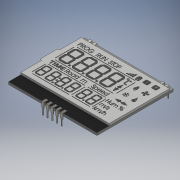
# Autodesk Inventor part: DF700543-05
Saved by Autodesk Inventor 2018 (Build 220112000, 112)
## iProperties
Created: 2018-02-18
Part Number: DF700543-05
Material: Generic
Document SubType Name: Modeling
Designer: danil
Density: 1 g/cm^3
Appearance: Default
Mass: 10.2861 g
Surface Area: 134.254 cm^2
Volume: 10.2861 cm^3
Author: danil
Autodesk Inventor part; units mm, degrees
(part 1 of 3)
ref_plane "YZ Plane" through (0, 0, 0) normal (1, 0, 0) x (0, 1, 0)
ref_plane "XZ Plane" through (0, 0, 0) normal (0, 1, 0) x (-1, 0, 0)
ref_plane "XY Plane" through (0, 0, 0) normal (0, 0, 1) x (1, 0, 0)
sketch "Sketch1" plane through (0, 0, 0) normal (0, 0, 1) x (1, 0, 0)
  line L0 (-23.765, -20.5) -> (23.765, -20.5)
  line L1 (23.765, -20.5) -> (23.765, 20.5)
  line L2 (23.765, 20.5) -> (-23.765, 20.5)
  line L3 (-23.765, 20.5) -> (-23.765, -20.5)
  line L4 (-23.765, -20.5) -> (23.765, 20.5) construction
  line L5 (23.765, -20.5) -> (-23.765, 20.5) construction
  arc A0 (-24.7705, -1.85) -> (-23.765, -2.75) centre (-23.865, -1.85) ccw
  arc A1 (-23.765, 7.25) -> (-24.7705, 6.35) centre (-23.865, 6.35) ccw
  line L6 (-24.7705, 6.35) -> (-24.7705, -1.85)
  point P0 (0, 0)
  point P1 (-24.765, -1.85)
  point P2 (-24.765, 6.35)
  dimension "d0" = 47.53
  dimension "d1" = 41
  constraints: 14 end point, 4 point on circle, 2 centre point, 2 coincident, 2 midpoint, 2 parallel, 2 point on line, 1 horizontal, 1 perpendicular
  measures "d0" distance of L2.end L1.end
  measures "d1" distance of L1.end L0.end
extrude "Extrusion1" add sketch "Sketch1" along normal blind 1.2
sketch "Sketch2" plane through (0, 0, 1.2) normal (0, 0, 1) x (1, 0, 0)
  line L0 (-23.765, 20.5) -> (-23.765, -20.5) projected
  line L1 (23.765, -20.5) -> (23.765, 20.5) projected
  line L2 (-23.765, 18.5) -> (23.765, 18.5)
  line L3 (23.765, 18.5) -> (23.765, -14)
  line L4 (23.765, -14) -> (-23.765, -14)
  line L5 (-23.765, -14) -> (-23.765, 18.5)
  arc A0 (-23.765, 7.25) -> (-24.7705, 6.35) centre (-23.865, 6.35) ccw projected
  line L6 (-24.7705, 6.35) -> (-24.7705, -1.85) projected
  arc A1 (-24.7705, -1.85) -> (-23.765, -2.75) centre (-23.865, -1.85) ccw projected
  line L7 (-23.765, -20.5) -> (23.765, -20.5) projected
  line L8 (23.765, 20.5) -> (-23.765, 20.5) projected
  dimension "d13" = 6.5
  dimension "d14" = 2
  constraints: 8 end point, 2 parallel, 2 point on line, 1 horizontal, 1 perpendicular
  measures "d13" distance between parallel lines of L4 L7
  measures "d14" distance between parallel lines of L8 L2
extrude "Extrusion2" add sketch "Sketch2" along normal blind 1.2 separate body contours L2 L1 L4 L0 | L0 A1 L6 A0
sketch "Sketch3" plane through (0, 0, 2.4) normal (0, 0, 1) x (1, 0, 0)
  line L0 (-19.2352, 12.1702) -> (-15.8959, 12.1702)
  line L1 (-15.8959, 12.1702) -> (-15.3617, 11.6361)
  line L2 (-15.3617, 11.6361) -> (-15.8375, 11.1603)
  line L3 (-15.8375, 11.1603) -> (-19.2759, 11.1603)
  line L4 (-19.2759, 11.1603) -> (-19.7605, 11.6449)
  line L5 (-19.7605, 11.6449) -> (-19.2352, 12.1702)
  line L6 (-19.8454, 11.56) -> (-19.3492, 11.0639)
  line L7 (-19.3492, 11.0639) -> (-19.3492, 7.616)
  line L8 (-19.3492, 7.616) -> (-19.8657, 7.0995)
  line L9 (-19.8657, 7.0995) -> (-20.3591, 7.5929)
  line L10 (-20.3591, 7.5929) -> (-20.3591, 11.0462)
  line L11 (-20.3591, 11.0462) -> (-19.8454, 11.56)
  line L12 (-15.2769, 11.5512) -> (-15.7818, 11.0462)
  line L13 (-15.7818, 11.0462) -> (-15.7818, 7.6242)
  line L14 (-15.7818, 7.6242) -> (-15.2572, 7.0995)
  line L15 (-15.2572, 7.0995) -> (-14.7719, 7.5848)
  line L16 (-14.7719, 7.5848) -> (-14.7719, 11.0462)
  line L17 (-14.7719, 11.0462) -> (-15.2769, 11.5512)
  line L18 (-19.7809, 7.0146) -> (-19.2759, 7.5196)
  line L19 (-19.2759, 7.5196) -> (-15.847, 7.5196)
  line L20 (-15.847, 7.5196) -> (-15.342, 7.0146)
  line L21 (-15.342, 7.0146) -> (-15.847, 6.5097)
  line L22 (-15.847, 6.5097) -> (-19.2759, 6.5097)
  line L23 (-19.2759, 6.5097) -> (-19.7809, 7.0146)
  line L24 (-19.8657, 6.9298) -> (-20.3591, 6.4364)
  line L25 (-20.3591, 6.4364) -> (-20.3591, 3.0156)
  line L26 (-20.3591, 3.0156) -> (-19.8379, 2.4943)
  line L27 (-19.8379, 2.4943) -> (-19.3492, 2.983)
  line L28 (-19.3492, 2.983) -> (-19.3492, 6.4133)
  line L29 (-19.3492, 6.4133) -> (-19.8657, 6.9298)
  line L30 (-19.753, 2.4095) -> (-19.2759, 1.9324)
  line L31 (-19.2759, 1.9324) -> (-15.847, 1.9324)
  line L32 (-15.847, 1.9324) -> (-15.3739, 2.4054)
  line L33 (-15.3739, 2.4054) -> (-15.9108, 2.9423)
  line L34 (-15.9108, 2.9423) -> (-19.2202, 2.9423)
  line L35 (-19.2202, 2.9423) -> (-19.753, 2.4095)
  line L36 (-15.2891, 2.4903) -> (-15.7818, 2.983)
  line L37 (-15.7818, 2.983) -> (-15.7818, 6.4051)
  line L38 (-15.7818, 6.4051) -> (-15.2572, 6.9298)
  line L39 (-15.2572, 6.9298) -> (-14.7719, 6.4445)
  line L40 (-14.7719, 6.4445) -> (-14.7719, 3.0075)
  line L41 (-14.7719, 3.0075) -> (-15.2891, 2.4903)
  line L42 (-14.3647, 2.8446) -> (-13.4606, 2.8446)
  line L43 (-13.4606, 2.8446) -> (-13.4606, 1.9405)
  line L44 (-13.4606, 1.9405) -> (-14.3647, 1.9405)
  line L45 (-14.3647, 1.9405) -> (-14.3647, 2.8446)
  line L46 (-7.9514, 7.0995) -> (-7.4661, 7.5848)
  line L47 (-8.0363, 7.0146) -> (-8.5412, 6.5097)
  line L48 (-7.4661, 7.5848) -> (-7.4661, 11.0462)
  line L49 (-8.4761, 11.0462) -> (-8.4761, 7.6242)
  line L50 (-7.4661, 11.0462) -> (-7.9711, 11.5512)
  line L51 (-8.056, 11.6361) -> (-8.5318, 11.1603)
  line L52 (-8.4761, 7.6242) -> (-7.9514, 7.0995)
  line L53 (-7.4661, 6.4445) -> (-7.4661, 3.0075)
  line L54 (-8.4761, 2.983) -> (-8.4761, 6.4051)
  line L55 (-8.6051, 2.9423) -> (-11.9145, 2.9423)
  line L56 (-11.9701, 1.9324) -> (-8.5412, 1.9324)
  line L57 (-12.4473, 2.4095) -> (-11.9701, 1.9324)
  line L58 (-11.9145, 2.9423) -> (-12.4473, 2.4095)
  line L59 (-12.5321, 2.4943) -> (-12.0434, 2.983)
  line L60 (-8.5412, 6.5097) -> (-11.9701, 6.5097)
  line L61 (-11.9701, 7.5196) -> (-8.5412, 7.5196)
  line L62 (-12.0434, 2.983) -> (-12.0434, 6.4133)
  line L63 (-11.9701, 6.5097) -> (-12.4751, 7.0146)
  line L64 (-12.4751, 7.0146) -> (-11.9701, 7.5196)
  line L65 (-13.0534, 6.4364) -> (-13.0534, 3.0156)
  line L66 (-13.0534, 3.0156) -> (-12.5321, 2.4943)
  line L67 (-8.4761, 6.4051) -> (-7.9514, 6.9298)
  line L68 (-8.5412, 7.5196) -> (-8.0363, 7.0146)
  line L69 (-7.9514, 6.9298) -> (-7.4661, 6.4445)
  line L70 (-8.0682, 2.4054) -> (-8.6051, 2.9423)
  line L71 (-8.5412, 1.9324) -> (-8.0682, 2.4054)
  line L72 (-7.4661, 3.0075) -> (-7.9833, 2.4903)
  line L73 (-7.9833, 2.4903) -> (-8.4761, 2.983)
  line L74 (-7.9711, 11.5512) -> (-8.4761, 11.0462)
  line L75 (-11.9294, 12.1702) -> (-8.5901, 12.1702)
  line L76 (-8.5901, 12.1702) -> (-8.056, 11.6361)
  line L77 (-8.5318, 11.1603) -> (-11.9701, 11.1603)
  line L78 (-11.9701, 11.1603) -> (-12.4547, 11.6449)
  line L79 (-12.4547, 11.6449) -> (-11.9294, 12.1702)
  line L80 (-12.5396, 11.56) -> (-12.0434, 11.0639)
  line L81 (-12.0434, 11.0639) -> (-12.0434, 7.616)
  line L82 (-12.0434, 7.616) -> (-12.56, 7.0995)
  line L83 (-12.56, 6.9298) -> (-13.0534, 6.4364)
  line L84 (-12.56, 7.0995) -> (-13.0534, 7.5929)
  line L85 (-13.0534, 7.5929) -> (-13.0534, 11.0462)
  line L86 (-13.0534, 11.0462) -> (-12.5396, 11.56)
  line L87 (-12.0434, 6.4133) -> (-12.56, 6.9298)
  line L88 (-0.6375, 7.0995) -> (-0.1522, 7.5848)
  line L89 (-0.7223, 7.0146) -> (-1.2273, 6.5097)
  line L90 (-0.1522, 7.5848) -> (-0.1522, 11.0462)
  line L91 (-1.1622, 11.0462) -> (-1.1622, 7.6242)
  line L92 (-0.1522, 11.0462) -> (-0.6572, 11.5512)
  line L93 (-0.742, 11.6361) -> (-1.2178, 11.1603)
  line L94 (-1.1622, 7.6242) -> (-0.6375, 7.0995)
  line L95 (-0.1522, 6.4445) -> (-0.1522, 3.0075)
  line L96 (-1.1622, 2.983) -> (-1.1622, 6.4051)
  line L97 (-1.2911, 2.9423) -> (-4.6005, 2.9423)
  line L98 (-4.6562, 1.9324) -> (-1.2273, 1.9324)
  line L99 (-5.1333, 2.4095) -> (-4.6562, 1.9324)
  line L100 (-4.6005, 2.9423) -> (-5.1333, 2.4095)
  line L101 (-5.2182, 2.4943) -> (-4.7295, 2.983)
  line L102 (-1.2273, 6.5097) -> (-4.6562, 6.5097)
  line L103 (-4.6562, 7.5196) -> (-1.2273, 7.5196)
  line L104 (-4.7295, 2.983) -> (-4.7295, 6.4133)
  line L105 (-4.6562, 6.5097) -> (-5.1612, 7.0146)
  line L106 (-5.1612, 7.0146) -> (-4.6562, 7.5196)
  line L107 (-5.7395, 6.4364) -> (-5.7395, 3.0156)
  line L108 (-5.7395, 3.0156) -> (-5.2182, 2.4943)
  line L109 (-1.1622, 6.4051) -> (-0.6375, 6.9298)
  line L110 (-1.2273, 7.5196) -> (-0.7223, 7.0146)
  line L111 (-0.6375, 6.9298) -> (-0.1522, 6.4445)
  line L112 (-0.7543, 2.4054) -> (-1.2911, 2.9423)
  line L113 (-1.2273, 1.9324) -> (-0.7543, 2.4054)
  line L114 (-0.1522, 3.0075) -> (-0.6694, 2.4903)
  line L115 (-0.6694, 2.4903) -> (-1.1622, 2.983)
  line L116 (-0.6572, 11.5512) -> (-1.1622, 11.0462)
  line L117 (-4.6155, 12.1702) -> (-1.2762, 12.1702)
  line L118 (-1.2762, 12.1702) -> (-0.742, 11.6361)
  line L119 (-1.2178, 11.1603) -> (-4.6562, 11.1603)
  line L120 (-4.6562, 11.1603) -> (-5.1408, 11.6449)
  line L121 (-5.1408, 11.6449) -> (-4.6155, 12.1702)
  line L122 (-5.2257, 11.56) -> (-4.7295, 11.0639)
  line L123 (-4.7295, 11.0639) -> (-4.7295, 7.616)
  line L124 (-4.7295, 7.616) -> (-5.246, 7.0995)
  line L125 (-5.246, 6.9298) -> (-5.7395, 6.4364)
  line L126 (-5.246, 7.0995) -> (-5.7395, 7.5929)
  line L127 (-5.7395, 7.5929) -> (-5.7395, 11.0462)
  line L128 (-5.7395, 11.0462) -> (-5.2257, 11.56)
  line L129 (-4.7295, 6.4133) -> (-5.246, 6.9298)
  line L130 (-7.0426, 2.8446) -> (-6.1386, 2.8446)
  line L131 (-6.1386, 2.8446) -> (-6.1386, 1.9405)
  line L132 (-6.1386, 1.9405) -> (-7.0426, 1.9405)
  line L133 (-7.0426, 1.9405) -> (-7.0426, 2.8446)
  line L134 (6.6113, 7.0995) -> (7.0965, 7.5848)
  line L135 (7.0965, 7.5848) -> (7.0965, 11.0462)
  line L136 (6.0866, 11.0462) -> (6.0866, 7.6242)
  line L137 (2.5925, 7.5196) -> (6.0214, 7.5196)
  line L138 (6.0866, 7.6242) -> (6.6113, 7.0995)
  line L139 (6.0214, 7.5196) -> (6.5264, 7.0146)
  line L140 (2.5192, 11.0639) -> (2.5192, 7.616)
  line L141 (1.5093, 7.5929) -> (1.5093, 11.0462)
  line L142 (2.5192, 7.616) -> (2.0027, 7.0995)
  line L143 (2.0876, 7.0146) -> (2.5925, 7.5196)
  line L144 (2.0027, 7.0995) -> (1.5093, 7.5929)
  line L145 (6.5264, 7.0146) -> (6.0214, 6.5097)
  line L146 (1.5093, 6.4364) -> (1.5093, 3.0156)
  line L147 (1.5093, 3.0156) -> (2.0306, 2.4943)
  line L148 (2.5192, 2.983) -> (2.5192, 6.4133)
  line L149 (6.0214, 6.5097) -> (2.5925, 6.5097)
  line L150 (2.0306, 2.4943) -> (2.5192, 2.983)
  line L151 (2.6482, 2.9423) -> (2.1154, 2.4095)
  line L152 (2.1154, 2.4095) -> (2.5925, 1.9324)
  line L153 (6.0866, 6.4051) -> (6.6113, 6.9298)
  line L154 (6.6113, 6.9298) -> (7.0965, 6.4445)
  line L155 (6.0866, 2.983) -> (6.0866, 6.4051)
  line L156 (7.0965, 6.4445) -> (7.0965, 3.0075)
  line L157 (2.5925, 1.9324) -> (6.0214, 1.9324)
  line L158 (5.9576, 2.9423) -> (2.6482, 2.9423)
  line L159 (2.0027, 6.9298) -> (1.5093, 6.4364)
  line L160 (2.5192, 6.4133) -> (2.0027, 6.9298)
  line L161 (2.5925, 6.5097) -> (2.0876, 7.0146)
  line L162 (1.5093, 11.0462) -> (2.0231, 11.56)
  line L163 (2.0231, 11.56) -> (2.5192, 11.0639)
  line L164 (2.5925, 11.1603) -> (2.1079, 11.6449)
  line L165 (6.0309, 11.1603) -> (2.5925, 11.1603)
  line L166 (7.0965, 11.0462) -> (6.5916, 11.5512)
  line L167 (6.5916, 11.5512) -> (6.0866, 11.0462)
  line L168 (6.5067, 11.6361) -> (6.0309, 11.1603)
  line L169 (5.9726, 12.1702) -> (6.5067, 11.6361)
  line L170 (2.6333, 12.1702) -> (5.9726, 12.1702)
  line L171 (2.1079, 11.6449) -> (2.6333, 12.1702)
  line L172 (6.4945, 2.4054) -> (5.9576, 2.9423)
  line L173 (6.0214, 1.9324) -> (6.4945, 2.4054)
  line L174 (6.5794, 2.4903) -> (6.0866, 2.983)
  line L175 (7.0965, 3.0075) -> (6.5794, 2.4903)
  line L176 (14.4675, 11.3639) -> (16.3084, 9.9795) construction
  line L177 (16.3084, 9.9795) -> (14.9887, 8.0409) construction
  spline S0 degree 2 poles (14.4675, 11.3639) (16.3084, 9.9795) (14.9887, 8.0409) knots 1 1 1 2 2 2
  line L178 (14.9887, 8.0409) -> (12.6861, 9.6083) construction
  line L179 (12.6861, 9.6083) -> (14.605, 9.7205) construction
  line L180 (14.605, 9.7205) -> (14.1661, 10.7205) construction
  spline S1 degree 3 poles (14.9887, 8.0409) (12.6861, 9.6083) (14.605, 9.7205) (14.1661, 10.7205) knots 1 1 1 1 2 2 2 2
  line L181 (14.1661, 10.7205) -> (14.3185, 10.6034) construction
  line L182 (14.3185, 10.6034) -> (14.4479, 10.478) construction
  spline S2 degree 2 poles (14.1661, 10.7205) (14.3185, 10.6034) (14.4479, 10.478) knots 1 1 1 2 2 2
  line L183 (14.4479, 10.478) -> (14.6135, 10.9014) construction
  line L184 (14.6135, 10.9014) -> (14.4675, 11.3639) construction
  spline S3 degree 2 poles (14.4479, 10.478) (14.6135, 10.9014) (14.4675, 11.3639) knots 1 1 1 2 2 2
  line L185 (14.7851, 10.077) -> (15.5699, 9.0537) construction
  line L186 (15.5699, 9.0537) -> (14.9652, 8.18) construction
  spline S4 degree 2 poles (14.7851, 10.077) (15.5699, 9.0537) (14.9652, 8.18) knots 1 1 1 2 2 2
  line L187 (14.9652, 8.18) -> (14.7161, 8.2775) construction
  line L188 (14.7161, 8.2775) -> (14.6139, 8.6034) construction
  spline S5 degree 2 poles (14.9652, 8.18) (14.7161, 8.2775) (14.6139, 8.6034) knots 1 1 1 2 2 2
  line L189 (14.7851, 10.077) -> (15.0718, 9.3642) construction
  line L190 (15.0718, 9.3642) -> (14.6139, 8.6034) construction
  spline S6 degree 2 poles (14.7851, 10.077) (15.0718, 9.3642) (14.6139, 8.6034) knots 1 1 1 2 2 2
  line L191 (14.5889, 8.6706) -> (14.5083, 8.8924) construction
  line L192 (14.5083, 8.8924) -> (14.6606, 9.2301) construction
  spline S7 degree 2 poles (14.5889, 8.6706) (14.5083, 8.8924) (14.6606, 9.2301) knots 1 1 1 2 2 2
  line L193 (14.6606, 9.2301) -> (14.6653, 8.8589) construction
  line L194 (14.6653, 8.8589) -> (14.5889, 8.6706) construction
  spline S8 degree 2 poles (14.6606, 9.2301) (14.6653, 8.8589) (14.5889, 8.6706) knots 1 1 1 2 2 2
  circle A0 centre (19.6475, 9.6698) radius 0.1249
  line L195 (19.1995, 11.1928) -> (19.5552, 11.232) construction
  line L196 (19.5552, 11.232) -> (19.7289, 10.9892) construction
  line L197 (19.7289, 10.9892) -> (19.8928, 10.7603) construction
  line L198 (19.8928, 10.7603) -> (19.8755, 10.4924) construction
  line L199 (19.8755, 10.4924) -> (19.8831, 10.2636) construction
  line L200 (19.8831, 10.2636) -> (19.8511, 10.134) construction
  line L201 (19.8511, 10.134) -> (19.7311, 9.7411) construction
  line L202 (19.7311, 9.7411) -> (19.338, 10.0526) construction
  line L203 (19.338, 10.0526) -> (19.1167, 10.2593) construction
  line L204 (19.1167, 10.2593) -> (18.8982, 10.4924) construction
  line L205 (18.8982, 10.4924) -> (18.6616, 10.8076) construction
  line L206 (18.6616, 10.8076) -> (18.9307, 11.0625) construction
  line L207 (18.9307, 11.0625) -> (19.034, 11.1603) construction
  line L208 (19.034, 11.1603) -> (19.1995, 11.1928) construction
  spline S9 degree 4 poles (19.1995, 11.1928) (19.5552, 11.232) (19.7289, 10.9892) (19.8928, 10.7603) (19.8755, 10.4924) (19.8831, 10.2636) (19.8511, 10.134) (19.7311, 9.7411) (19.338, 10.0526) (19.1167, 10.2593) (18.8982, 10.4924) (18.6616, 10.8076) (18.9307, 11.0625) (19.034, 11.1603) (19.1995, 11.1928) knots 1 1 1 1 1 2 3 4 5 6 7 8 9 10 11 12 12 12 12 12
  line L209 (19.2647, 9.3603) -> (19.058, 9.1391) construction
  line L210 (18.1244, 9.2218) -> (18.0853, 9.5775) construction
  line L211 (18.157, 9.0563) -> (18.1244, 9.2218) construction
  line L212 (18.2547, 8.9531) -> (18.157, 9.0563) construction
  line L213 (18.0853, 9.5775) -> (18.328, 9.7512) construction
  line L214 (18.5097, 8.6839) -> (18.2547, 8.9531) construction
  line L215 (18.328, 9.7512) -> (18.557, 9.9151) construction
  line L216 (18.557, 9.9151) -> (18.8249, 9.8978) construction
  line L217 (18.8249, 8.9205) -> (18.5097, 8.6839) construction
  line L218 (18.8249, 9.8978) -> (19.0537, 9.9055) construction
  line L219 (19.058, 9.1391) -> (18.8249, 8.9205) construction
  line L220 (19.0537, 9.9055) -> (19.1832, 9.8734) construction
  spline S10 degree 4 poles (18.1244, 9.2218) (18.0853, 9.5775) (18.328, 9.7512) (18.557, 9.9151) (18.8249, 9.8978) (19.0537, 9.9055) (19.1832, 9.8734) (19.5762, 9.7534) (19.2647, 9.3603) (19.058, 9.1391) (18.8249, 8.9205) (18.5097, 8.6839) (18.2547, 8.9531) (18.157, 9.0563) (18.1244, 9.2218) knots 1 1 1 1 1 2 3 4 5 6 7 8 9 10 11 12 12 12 12 12
  line L221 (19.1832, 9.8734) -> (19.5762, 9.7534) construction
  line L222 (19.5762, 9.7534) -> (19.2647, 9.3603) construction
  line L223 (19.957, 9.287) -> (20.1782, 9.0803) construction
  line L224 (20.0954, 8.1467) -> (19.7398, 8.1076) construction
  line L225 (20.261, 8.1793) -> (20.0954, 8.1467) construction
  line L226 (20.3642, 8.2771) -> (20.261, 8.1793) construction
  line L227 (19.7398, 8.1076) -> (19.566, 8.3504) construction
  line L228 (20.6334, 8.532) -> (20.3642, 8.2771) construction
  line L229 (19.566, 8.3504) -> (19.4022, 8.5793) construction
  line L230 (19.4022, 8.5793) -> (19.4194, 8.8472) construction
  line L231 (20.3968, 8.8472) -> (20.6334, 8.532) construction
  line L232 (19.4194, 8.8472) -> (19.4118, 9.076) construction
  line L233 (20.1782, 9.0803) -> (20.3968, 8.8472) construction
  line L234 (19.4118, 9.076) -> (19.4439, 9.2055) construction
  spline S11 degree 4 poles (20.0954, 8.1467) (19.7398, 8.1076) (19.566, 8.3504) (19.4022, 8.5793) (19.4194, 8.8472) (19.4118, 9.076) (19.4439, 9.2055) (19.5638, 9.5985) (19.957, 9.287) (20.1782, 9.0803) (20.3968, 8.8472) (20.6334, 8.532) (20.3642, 8.2771) (20.261, 8.1793) (20.0954, 8.1467) knots 1 1 1 1 1 2 3 4 5 6 7 8 9 10 11 12 12 12 12 12
  line L235 (19.4439, 9.2055) -> (19.5638, 9.5985) construction
  line L236 (19.5638, 9.5985) -> (19.957, 9.287) construction
  line L237 (20.0303, 9.9793) -> (20.237, 10.2005) construction
  line L238 (21.1705, 10.1178) -> (21.2097, 9.7621) construction
  line L239 (21.138, 10.2833) -> (21.1705, 10.1178) construction
  line L240 (21.0402, 10.3865) -> (21.138, 10.2833) construction
  line L241 (21.2097, 9.7621) -> (20.9669, 9.5883) construction
  line L242 (20.7853, 10.6557) -> (21.0402, 10.3865) construction
  line L243 (20.9669, 9.5883) -> (20.738, 9.4245) construction
  line L244 (20.738, 9.4245) -> (20.4701, 9.4417) construction
  line L245 (20.4701, 10.4191) -> (20.7853, 10.6557) construction
  line L246 (20.4701, 9.4417) -> (20.2413, 9.4341) construction
  line L247 (20.237, 10.2005) -> (20.4701, 10.4191) construction
  line L248 (20.2413, 9.4341) -> (20.1117, 9.4662) construction
  spline S12 degree 4 poles (21.1705, 10.1178) (21.2097, 9.7621) (20.9669, 9.5883) (20.738, 9.4245) (20.4701, 9.4417) (20.2413, 9.4341) (20.1117, 9.4662) (19.7188, 9.5862) (20.0303, 9.9793) (20.237, 10.2005) (20.4701, 10.4191) (20.7853, 10.6557) (21.0402, 10.3865) (21.138, 10.2833) (21.1705, 10.1178) knots 1 1 1 1 1 2 3 4 5 6 7 8 9 10 11 12 12 12 12 12
  line L249 (20.1117, 9.4662) -> (19.7188, 9.5862) construction
  line L250 (19.7188, 9.5862) -> (20.0303, 9.9793) construction
  line L251 (19.5497, 5.7196) -> (19.5647, 4.7442) construction
  line L252 (19.5647, 4.7442) -> (18.8057, 3.7702) construction
  line L253 (18.8057, 3.7702) -> (18.6673, 3.0699) construction
  line L254 (18.6673, 3.0699) -> (19.1185, 2.563) construction
  line L255 (19.1185, 2.563) -> (19.6335, 2.4054) construction
  line L256 (19.6335, 2.4054) -> (20.1503, 2.563) construction
  line L257 (20.1503, 2.563) -> (20.738, 3.016) construction
  line L258 (20.738, 3.016) -> (20.5746, 4.0414) construction
  line L259 (20.5746, 4.0414) -> (20.14, 4.3215) construction
  line L260 (20.14, 4.3215) -> (19.5497, 5.7196) construction
  spline S13 degree 4 poles (19.5497, 5.7196) (19.5647, 4.7442) (18.8057, 3.7702) (18.6673, 3.0699) (19.1185, 2.563) (19.6335, 2.4054) (20.1503, 2.563) (20.738, 3.016) (20.5746, 4.0414) (20.14, 4.3215) (19.5497, 5.7196) knots 1 1 1 1 1 2 3 4 5 6 7 8 8 8 8 8
  line L261 (19.9488, 4.0988) -> (20.2922, 3.6032) construction
  line L262 (20.2922, 3.6032) -> (20.0384, 2.8283) construction
  spline S14 degree 2 poles (19.9488, 4.0988) (20.2922, 3.6032) (20.0384, 2.8283) knots 1 1 1 2 2 2
  line L263 (19.9488, 4.0988) -> (20.482, 3.8976) construction
  line L264 (20.482, 3.8976) -> (20.6648, 3.3088) construction
  line L265 (20.6648, 3.3088) -> (20.0384, 2.8283) construction
  spline S15 degree 3 poles (19.9488, 4.0988) (20.482, 3.8976) (20.6648, 3.3088) (20.0384, 2.8283) knots 1 1 1 1 2 2 2 2
  line L266 (-20.7582, 16.0471) -> (-21.3039, 16.0471)
  line L267 (-21.3039, 16.0471) -> (-21.3039, 13.8562)
  line L268 (-21.3039, 13.8562) -> (-21.0922, 13.8562)
  line L269 (-21.0922, 13.8562) -> (-21.0922, 14.7765)
  line L270 (-21.0922, 14.7765) -> (-20.6524, 14.7765)
  line L271 (-20.6686, 14.9964) -> (-21.0922, 14.9964)
  line L272 (-21.0922, 14.9964) -> (-21.0922, 15.8272)
  line L273 (-21.0922, 15.8272) -> (-20.6768, 15.8272)
  line L274 (-20.7582, 16.0471) -> (-20.3847, 16.0471) construction
  line L275 (-20.3847, 16.0471) -> (-20.207, 15.8522) construction
  line L276 (-20.207, 15.8522) -> (-20.0265, 15.654) construction
  line L277 (-20.0265, 15.654) -> (-20.0128, 15.1057) construction
  line L278 (-20.0128, 15.1057) -> (-20.3862, 14.7765) construction
  line L279 (-20.3862, 14.7765) -> (-20.6524, 14.7765) construction
  spline S16 degree 4 poles (-20.7582, 16.0471) (-20.3847, 16.0471) (-20.207, 15.8522) (-20.0265, 15.654) (-20.0128, 15.1057) (-20.3862, 14.7765) (-20.6524, 14.7765) knots 0 0 0 0 0 1 2 3 3 3 3 3
  line L280 (-20.6768, 15.8272) -> (-20.4466, 15.8272) construction
  line L281 (-20.4466, 15.8272) -> (-20.2505, 15.6009) construction
  line L282 (-20.2505, 15.6009) -> (-20.184, 15.1773) construction
  line L283 (-20.184, 15.1773) -> (-20.5329, 14.9964) construction
  line L284 (-20.5329, 14.9964) -> (-20.6686, 14.9964) construction
  spline S17 degree 4 poles (-20.6768, 15.8272) (-20.4466, 15.8272) (-20.2505, 15.6009) (-20.184, 15.1773) (-20.5329, 14.9964) (-20.6686, 14.9964) knots 0 0 0 0 0 1 2 2 2 2 2
  line L285 (0.1003, 14.9964) -> (-0.1848, 14.9964)
  line L286 (0.3782, 14.9964) -> (0.1003, 14.9964) construction
  spline S18 degree 4 poles (0.0476, 15.8353) (0.3396, 15.8353) (0.6092, 15.7213) (0.6606, 15.2454) (0.3782, 14.9964) (0.1003, 14.9964) knots 0 0 0 0 0 1 2 2 2 2 2
  line L287 (0.0476, 15.8353) -> (0.3396, 15.8353) construction
  line L288 (0.3396, 15.8353) -> (0.6092, 15.7213) construction
  line L289 (0.6092, 15.7213) -> (0.6606, 15.2454) construction
  line L290 (0.6606, 15.2454) -> (0.3782, 14.9964) construction
  line L291 (0.4494, 14.7765) -> (0.0758, 14.7765) construction
  spline S19 degree 4 poles (0.198, 16.0471) (0.4509, 16.0471) (0.7076, 15.8409) (0.8419, 15.5088) (0.7445, 15.0251) (0.4494, 14.7765) (0.0758, 14.7765) knots 0 0 0 0 0 1 2 3 3 3 3 3
  line L292 (0.198, 16.0471) -> (0.4509, 16.0471) construction
  line L293 (0.4509, 16.0471) -> (0.7076, 15.8409) construction
  line L294 (0.7076, 15.8409) -> (0.8419, 15.5088) construction
  line L295 (0.8419, 15.5088) -> (0.7445, 15.0251) construction
  line L296 (0.7445, 15.0251) -> (0.4494, 14.7765) construction
  line L297 (-0.1848, 15.8353) -> (0.0476, 15.8353)
  line L298 (-0.1848, 14.9964) -> (-0.1848, 15.8353)
  line L299 (-0.3803, 16.0471) -> (-0.3803, 13.8562)
  line L300 (0.198, 16.0471) -> (-0.3803, 16.0471)
  line L301 (-0.1848, 13.8562) -> (-0.1848, 14.7765)
  line L302 (-0.3803, 13.8562) -> (-0.1848, 13.8562)
  line L303 (-0.1848, 14.7765) -> (0.0758, 14.7765)
  line L304 (-19.1537, 16.0471) -> (-18.7709, 16.0471) construction
  line L305 (-18.7709, 16.0471) -> (-18.3972, 15.6009) construction
  line L306 (-18.3972, 15.6009) -> (-18.4491, 15.2045) construction
  line L307 (-18.4491, 15.2045) -> (-18.5937, 14.7949) construction
  line L308 (-18.5937, 14.7949) -> (-18.8319, 14.7415) construction
  line L309 (-18.8319, 14.7415) -> (-18.9664, 14.7113) construction
  spline S20 degree 4 poles (-19.1537, 16.0471) (-18.7709, 16.0471) (-18.3972, 15.6009) (-18.4491, 15.2045) (-18.5937, 14.7949) (-18.8319, 14.7415) (-18.9664, 14.7113) knots 1 1 1 1 1 2 3 4 4 4 4 4
  line L310 (-19.1049, 15.8272) -> (-18.8991, 15.8272) construction
  line L311 (-18.8991, 15.8272) -> (-18.694, 15.5708) construction
  line L312 (-18.694, 15.5708) -> (-18.6707, 15.4194) construction
  line L313 (-18.6707, 15.4194) -> (-18.6819, 15.2454) construction
  line L314 (-18.6819, 15.2454) -> (-18.7508, 15.0251) construction
  line L315 (-18.7508, 15.0251) -> (-18.9696, 14.9068) construction
  line L316 (-18.9696, 14.9068) -> (-19.1293, 14.9068) construction
  spline S21 degree 4 poles (-19.1049, 15.8272) (-18.8991, 15.8272) (-18.694, 15.5708) (-18.6707, 15.4194) (-18.6819, 15.2454) (-18.7508, 15.0251) (-18.9696, 14.9068) (-19.1293, 14.9068) knots 1 1 1 1 1 2 3 4 5 5 5 5 5
  line L317 (-19.1537, 16.0471) -> (-19.8053, 16.0471)
  line L318 (-19.8053, 16.0471) -> (-19.8053, 13.8562)
  line L319 (-19.8053, 13.8562) -> (-19.6017, 13.8562)
  line L320 (-19.6017, 13.8562) -> (-19.6017, 15.8272)
  line L321 (-19.6017, 15.8272) -> (-19.1049, 15.8272)
  line L322 (-19.1293, 14.9068) -> (-19.3329, 14.9068)
  line L323 (-19.3329, 14.9068) -> (-18.7058, 13.8562)
  line L324 (-18.7058, 13.8562) -> (-18.4614, 13.8562)
  line L325 (-18.4614, 13.8562) -> (-18.9664, 14.7113)
  line L326 (-10.4866, 16.0471) -> (-10.1128, 15.6009) construction
  spline S22 degree 4 poles (-10.8694, 16.0471) (-10.4866, 16.0471) (-10.1128, 15.6009) (-10.1648, 15.2045) (-10.3094, 14.7949) (-10.5475, 14.7415) (-10.6821, 14.7113) knots 1 1 1 1 1 2 3 4 4 4 4 4
  line L327 (-10.8694, 16.0471) -> (-10.4866, 16.0471) construction
  line L328 (-10.1128, 15.6009) -> (-10.1648, 15.2045) construction
  line L329 (-10.1648, 15.2045) -> (-10.3094, 14.7949) construction
  line L330 (-10.3094, 14.7949) -> (-10.5475, 14.7415) construction
  line L331 (-10.5475, 14.7415) -> (-10.6821, 14.7113) construction
  line L332 (-10.4096, 15.5708) -> (-10.3864, 15.4194) construction
  spline S23 degree 4 poles (-10.8205, 15.8272) (-10.6148, 15.8272) (-10.4096, 15.5708) (-10.3864, 15.4194) (-10.3975, 15.2454) (-10.4664, 15.0251) (-10.6852, 14.9068) (-10.845, 14.9068) knots 1 1 1 1 1 2 3 4 5 5 5 5 5
  line L333 (-10.8205, 15.8272) -> (-10.6148, 15.8272) construction
  line L334 (-10.6148, 15.8272) -> (-10.4096, 15.5708) construction
  line L335 (-10.3864, 15.4194) -> (-10.3975, 15.2454) construction
  line L336 (-10.3975, 15.2454) -> (-10.4664, 15.0251) construction
  line L337 (-10.4664, 15.0251) -> (-10.6852, 14.9068) construction
  line L338 (-10.6852, 14.9068) -> (-10.845, 14.9068) construction
  line L339 (-10.8694, 16.0471) -> (-11.521, 16.0471)
  line L340 (-10.845, 14.9068) -> (-11.0486, 14.9068)
  line L341 (-11.3173, 15.8272) -> (-10.8205, 15.8272)
  line L342 (-10.1771, 13.8562) -> (-10.6821, 14.7113)
  line L343 (-10.4214, 13.8562) -> (-10.1771, 13.8562)
  line L344 (-11.0486, 14.9068) -> (-10.4214, 13.8562)
  line L345 (-11.521, 13.8562) -> (-11.3173, 13.8562)
  line L346 (-11.3173, 13.8562) -> (-11.3173, 15.8272)
  line L347 (-11.521, 16.0471) -> (-11.521, 13.8562)
  line L348 (-11.4326, 0.2627) -> (-11.0588, -0.1834) construction
  spline S24 degree 4 poles (-11.8154, 0.2627) (-11.4326, 0.2627) (-11.0588, -0.1834) (-11.1108, -0.5799) (-11.2554, -0.9895) (-11.4935, -1.0429) (-11.6281, -1.073) knots 1 1 1 1 1 2 3 4 4 4 4 4
  line L349 (-11.8154, 0.2627) -> (-11.4326, 0.2627) construction
  line L350 (-11.0588, -0.1834) -> (-11.1108, -0.5799) construction
  line L351 (-11.1108, -0.5799) -> (-11.2554, -0.9895) construction
  line L352 (-11.2554, -0.9895) -> (-11.4935, -1.0429) construction
  line L353 (-11.4935, -1.0429) -> (-11.6281, -1.073) construction
  line L354 (-11.3556, -0.2136) -> (-11.3324, -0.3649) construction
  spline S25 degree 4 poles (-11.7665, 0.0428) (-11.5608, 0.0428) (-11.3556, -0.2136) (-11.3324, -0.3649) (-11.3435, -0.539) (-11.4124, -0.7593) (-11.6312, -0.8776) (-11.791, -0.8776) knots 1 1 1 1 1 2 3 4 5 5 5 5 5
  line L355 (-11.7665, 0.0428) -> (-11.5608, 0.0428) construction
  line L356 (-11.5608, 0.0428) -> (-11.3556, -0.2136) construction
  line L357 (-11.3324, -0.3649) -> (-11.3435, -0.539) construction
  line L358 (-11.3435, -0.539) -> (-11.4124, -0.7593) construction
  line L359 (-11.4124, -0.7593) -> (-11.6312, -0.8776) construction
  line L360 (-11.6312, -0.8776) -> (-11.791, -0.8776) construction
  line L361 (-11.8154, 0.2627) -> (-12.467, 0.2627)
  line L362 (-11.791, -0.8776) -> (-11.9946, -0.8776)
  line L363 (-12.2633, 0.0428) -> (-11.7665, 0.0428)
  line L364 (-11.1231, -1.9282) -> (-11.6281, -1.073)
  line L365 (-11.3674, -1.9282) -> (-11.1231, -1.9282)
  line L366 (-11.9946, -0.8776) -> (-11.3674, -1.9282)
  line L367 (-12.467, -1.9282) -> (-12.2633, -1.9282)
  line L368 (-12.2633, -1.9282) -> (-12.2633, 0.0428)
  line L369 (-12.467, 0.2627) -> (-12.467, -1.9282)
  ellipse E0 centre (-17.1528, 14.9561) end of major axis (-17.1552, 15.8894) minor radius 0.8681
  ellipse E1 centre (-17.1528, 14.9561) end of major axis (-17.1558, 16.1072) minor radius 1.0859
  ellipse E2 centre (-1.6325, 14.9516) end of major axis (-1.635, 15.8849) minor radius 0.7864
  ellipse E3 centre (-1.6325, 14.9516) end of major axis (-1.6355, 16.1027) minor radius 1.0034
  ellipse E4 centre (-10.1377, -1.0984) end of major axis (-10.1377, -0.421) minor radius 0.6048
  ellipse E5 centre (-10.1377, -1.0984) end of major axis (-10.1377, -0.2081) minor radius 0.8274
  ellipse E6 centre (-14.8138, 14.964) end of major axis (-14.8138, 15.8973) minor radius 0.8681 (-14.0972, 15.4908) -> (-13.9781, 14.7113) ccw
  ellipse E7 centre (-14.8138, 14.964) end of major axis (-14.8138, 16.1154) minor radius 1.0862 (-13.848, 15.4908) -> (-13.729, 14.9068) ccw
  line L370 (-15.0488, 14.9068) -> (-13.729, 14.9068)
  line L371 (-15.0488, 14.9068) -> (-15.0488, 14.7113)
  line L372 (-15.0488, 14.7113) -> (-13.9781, 14.7113)
  line L373 (-14.0972, 15.4908) -> (-13.848, 15.4908)
  line L374 (-9.8525, 14.5566) -> (-9.8525, 14.1399) construction
  line L375 (-8.5086, 14.1529) -> (-8.5086, 14.5647) construction
  spline S26 degree 4 poles (-9.8525, 14.5566) (-9.8525, 14.1399) (-9.4835, 13.6893) (-8.8106, 13.708) (-8.5086, 14.1529) (-8.5086, 14.5647) knots 0 0 0 0 0 0.493568 1 1 1 1 1
  line L376 (-9.6489, 14.6706) -> (-9.6489, 14.1851) construction
  line L377 (-9.6489, 14.1851) -> (-9.3769, 13.9732) construction
  line L378 (-9.3769, 13.9732) -> (-8.9647, 13.9732) construction
  line L379 (-8.9647, 13.9732) -> (-8.7123, 14.2124) construction
  line L380 (-8.7123, 14.2124) -> (-8.7123, 14.6299) construction
  spline S27 degree 4 poles (-9.6489, 14.6706) (-9.6489, 14.1851) (-9.3769, 13.9732) (-8.9647, 13.9732) (-8.7123, 14.2124) (-8.7123, 14.6299) knots 1 1 1 1 1 2 3 3 3 3 3
  line L381 (-9.8525, 14.1399) -> (-9.4835, 13.6893) construction
  line L382 (-9.4835, 13.6893) -> (-8.8106, 13.708) construction
  line L383 (-8.8106, 13.708) -> (-8.5086, 14.1529) construction
  line L384 (-9.8525, 14.5566) -> (-9.8525, 16.0552)
  line L385 (-9.8525, 16.0552) -> (-9.6489, 16.0552)
  line L386 (-9.6489, 16.0552) -> (-9.6489, 14.6706)
  line L387 (-8.7123, 14.6299) -> (-8.7123, 16.0552)
  line L388 (-8.7123, 16.0552) -> (-8.5086, 16.0552)
  line L389 (-8.5086, 16.0552) -> (-8.5086, 14.5647)
  line L390 (-8.1503, 13.8643) -> (-7.9467, 13.8643)
  line L391 (-7.9467, 13.8643) -> (-7.9711, 15.8027)
  line L392 (-7.9711, 15.8027) -> (-6.8064, 13.8643)
  line L393 (-6.8064, 13.8643) -> (-6.5621, 13.8643)
  line L394 (-6.5621, 13.8643) -> (-6.5621, 16.0552)
  line L395 (-6.5621, 16.0552) -> (-6.7657, 16.0552)
  line L396 (-6.7657, 16.0552) -> (-6.7413, 14.1249)
  line L397 (-6.7413, 14.1249) -> (-7.8978, 16.0552)
  line L398 (-7.8978, 16.0552) -> (-8.1503, 16.0552)
  line L399 (-8.1503, 16.0552) -> (-8.1503, 13.8643)
  line L400 (0.198, 2.8446) -> (1.1021, 2.8446)
  line L401 (1.1021, 2.8446) -> (1.1021, 1.9405)
  line L402 (1.1021, 1.9405) -> (0.198, 1.9405)
  line L403 (0.198, 1.9405) -> (0.198, 2.8446)
  line L404 (-3.9476, 15.5095) -> (-3.9779, 15.7806) construction
  line L405 (-3.9779, 15.7806) -> (-4.1862, 15.9252) construction
  line L406 (-4.1862, 15.9252) -> (-4.4043, 15.8849) construction
  line L407 (-4.4043, 15.8849) -> (-4.5739, 15.7142) construction
  line L408 (-4.5739, 15.7142) -> (-4.6302, 15.4194) construction
  line L409 (-4.6302, 15.4194) -> (-4.4593, 15.1621) construction
  line L410 (-4.4593, 15.1621) -> (-4.0723, 15.11) construction
  line L411 (-4.0723, 15.11) -> (-3.8582, 14.9588) construction
  line L412 (-3.8582, 14.9588) -> (-3.6853, 14.6916) construction
  line L413 (-3.6853, 14.6916) -> (-3.7264, 14.2862) construction
  line L414 (-3.7264, 14.2862) -> (-3.8904, 13.889) construction
  line L415 (-3.8904, 13.889) -> (-4.2658, 13.7493) construction
  line L416 (-4.2658, 13.7493) -> (-4.7068, 13.8784) construction
  line L417 (-4.7068, 13.8784) -> (-4.8227, 14.2261) construction
  line L418 (-4.8227, 14.2261) -> (-4.8354, 14.4833) construction
  spline S28 degree 4 poles (-3.9476, 15.5095) (-3.9779, 15.7806) (-4.1862, 15.9252) (-4.4043, 15.8849) (-4.5739, 15.7142) (-4.6302, 15.4194) (-4.4593, 15.1621) (-4.0723, 15.11) (-3.8582, 14.9588) (-3.6853, 14.6916) (-3.7264, 14.2862) (-3.8904, 13.889) (-4.2658, 13.7493) (-4.7068, 13.8784) (-4.8227, 14.2261) (-4.8354, 14.4833) knots 1 1 1 1 1 2 3 4 5 6 7 8 9 10 11 12 13 13 13 13 13
  line L419 (-4.6481, 14.4833) -> (-4.6412, 14.2657) construction
  line L420 (-4.6412, 14.2657) -> (-4.4914, 14.0331) construction
  line L421 (-4.4914, 14.0331) -> (-4.1935, 14.0064) construction
  line L422 (-4.1935, 14.0064) -> (-3.978, 14.1529) construction
  line L423 (-3.978, 14.1529) -> (-3.8904, 14.4212) construction
  line L424 (-3.8904, 14.4212) -> (-3.9271, 14.6398) construction
  line L425 (-3.9271, 14.6398) -> (-4.0347, 14.7996) construction
  line L426 (-4.0347, 14.7996) -> (-4.2657, 14.9111) construction
  line L427 (-4.2657, 14.9111) -> (-4.5552, 15.0147) construction
  line L428 (-4.5552, 15.0147) -> (-4.7685, 15.223) construction
  line L429 (-4.7685, 15.223) -> (-4.796, 15.4908) construction
  line L430 (-4.796, 15.4908) -> (-4.7685, 15.7622) construction
  line L431 (-4.7685, 15.7622) -> (-4.6273, 15.9725) construction
  line L432 (-4.6273, 15.9725) -> (-4.3975, 16.1191) construction
  line L433 (-4.3975, 16.1191) -> (-4.0397, 16.0968) construction
  line L434 (-4.0397, 16.0968) -> (-3.8663, 15.9357) construction
  line L435 (-3.8663, 15.9357) -> (-3.7749, 15.6941) construction
  line L436 (-3.7749, 15.6941) -> (-3.7603, 15.5095) construction
  spline S29 degree 4 poles (-4.6481, 14.4833) (-4.6412, 14.2657) (-4.4914, 14.0331) (-4.1935, 14.0064) (-3.978, 14.1529) (-3.8904, 14.4212) (-3.9271, 14.6398) (-4.0347, 14.7996) (-4.2657, 14.9111) (-4.5552, 15.0147) (-4.7685, 15.223) (-4.796, 15.4908) (-4.7685, 15.7622) (-4.6273, 15.9725) (-4.3975, 16.1191) (-4.0397, 16.0968) (-3.8663, 15.9357) (-3.7749, 15.6941) (-3.7603, 15.5095) knots 1 1 1 1 1 2 3 4 5 6 7 8 9 10 11 12 13 14 15 16 16 16 16 16
  line L437 (-3.9476, 15.5095) -> (-3.7603, 15.5095)
  line L438 (-4.8354, 14.4833) -> (-4.6481, 14.4833)
  line L439 (-2.6282, 15.8353) -> (-3.0273, 15.8353)
  line L440 (-3.0273, 15.8353) -> (-3.0273, 13.8562)
  line L441 (-3.0273, 13.8562) -> (-3.2146, 13.8562)
  line L442 (-3.2146, 13.8562) -> (-3.2146, 15.8353)
  line L443 (-3.2146, 15.8353) -> (-3.6137, 15.8353)
  line L444 (-3.6137, 15.8353) -> (-3.6137, 16.0471)
  line L445 (-3.6137, 16.0471) -> (-2.6282, 16.0471)
  line L446 (-2.6282, 16.0471) -> (-2.6282, 15.8353)
  line L447 (1.7326, -1.872) -> (1.603, -1.525) construction
  spline S30 degree 4 poles (2.5437, -0.2504) (2.5126, 0.0286) (2.3056, 0.1473) (2.0629, 0.1359) (1.8645, -0.0436) (1.807, -0.3872) (2.0453, -0.5883) (2.4154, -0.6823) (2.6464, -0.7917) (2.8192, -1.0588) (2.7684, -1.5443) (2.5839, -1.872) (2.1736, -2.0012) (1.7326, -1.872) (1.603, -1.525) (1.5907, -1.2766) knots 1 1 1 1 1 2 3 4 5 6 7 8 9 10 11 12 13 13 13 13 13
  line L448 (2.5437, -0.2504) -> (2.5126, 0.0286) construction
  line L449 (2.5126, 0.0286) -> (2.3056, 0.1473) construction
  line L450 (2.3056, 0.1473) -> (2.0629, 0.1359) construction
  line L451 (2.0629, 0.1359) -> (1.8645, -0.0436) construction
  line L452 (1.8645, -0.0436) -> (1.807, -0.3872) construction
  line L453 (1.807, -0.3872) -> (2.0453, -0.5883) construction
  line L454 (2.0453, -0.5883) -> (2.4154, -0.6823) construction
  line L455 (2.4154, -0.6823) -> (2.6464, -0.7917) construction
  line L456 (2.6464, -0.7917) -> (2.8192, -1.0588) construction
  line L457 (2.8192, -1.0588) -> (2.7684, -1.5443) construction
  line L458 (2.7684, -1.5443) -> (2.5839, -1.872) construction
  line L459 (2.5839, -1.872) -> (2.1736, -2.0012) construction
  line L460 (2.1736, -2.0012) -> (1.7326, -1.872) construction
  line L461 (1.603, -1.525) -> (1.5907, -1.2766) construction
  line L462 (1.5907, -1.2766) -> (1.7862, -1.2766)
  line L463 (2.5437, -0.2504) -> (2.7391, -0.2504)
  line L464 (2.7427, -0.0223) -> (2.7391, -0.2504) construction
  spline S31 degree 4 poles (1.7862, -1.2766) (1.7931, -1.4943) (1.9429, -1.7268) (2.2408, -1.7536) (2.5007, -1.6259) (2.5925, -1.3855) (2.5839, -1.0984) (2.4194, -0.9386) (2.1686, -0.8488) (1.8791, -0.7453) (1.6658, -0.537) (1.6383, -0.2692) (1.6658, 0.0022) (1.807, 0.2125) (2.0368, 0.3592) (2.3946, 0.3368) (2.5925, 0.2184) (2.7427, -0.0223) (2.7391, -0.2504) knots 1 1 1 1 1 2 3 4 5 6 7 8 9 10 11 12 13 14 15 16 16 16 16 16
  line L465 (1.7862, -1.2766) -> (1.7931, -1.4943) construction
  line L466 (1.7931, -1.4943) -> (1.9429, -1.7268) construction
  line L467 (1.9429, -1.7268) -> (2.2408, -1.7536) construction
  line L468 (2.2408, -1.7536) -> (2.5007, -1.6259) construction
  line L469 (2.5007, -1.6259) -> (2.5925, -1.3855) construction
  line L470 (2.5925, -1.3855) -> (2.5839, -1.0984) construction
  line L471 (2.5839, -1.0984) -> (2.4194, -0.9386) construction
  line L472 (2.4194, -0.9386) -> (2.1686, -0.8488) construction
  line L473 (2.1686, -0.8488) -> (1.8791, -0.7453) construction
  line L474 (1.8791, -0.7453) -> (1.6658, -0.537) construction
  line L475 (1.6658, -0.537) -> (1.6383, -0.2692) construction
  line L476 (1.6383, -0.2692) -> (1.6658, 0.0022) construction
  line L477 (1.6658, 0.0022) -> (1.807, 0.2125) construction
  line L478 (1.807, 0.2125) -> (2.0368, 0.3592) construction
  line L479 (2.0368, 0.3592) -> (2.3946, 0.3368) construction
  line L480 (2.3946, 0.3368) -> (2.5925, 0.2184) construction
  line L481 (2.5925, 0.2184) -> (2.7427, -0.0223) construction
  line L482 (-14.2099, -0.169) -> (-14.5271, -0.169) construction
  line L483 (-14.5271, -0.169) -> (-14.6742, -0.4031) construction
  line L484 (-14.6742, -0.4031) -> (-14.6742, -0.6576) construction
  spline S32 degree 3 poles (-14.2099, -0.169) (-14.5271, -0.169) (-14.6742, -0.4031) (-14.6742, -0.6576) knots 1 1 1 1 2 2 2 2
  line L485 (-14.6742, -1.0242) -> (-14.6742, -1.4358) construction
  line L486 (-14.6742, -1.4358) -> (-14.4564, -1.5454) construction
  line L487 (-14.4564, -1.5454) -> (-14.2344, -1.5454) construction
  spline S33 degree 3 poles (-14.6742, -1.0242) (-14.6742, -1.4358) (-14.4564, -1.5454) (-14.2344, -1.5454) knots 1 1 1 1 2 2 2 2
  line L488 (-14.6742, -1.0242) -> (-13.371, -1.0242)
  line L489 (-13.371, -1.0242) -> (-13.371, -0.6576)
  line L490 (-13.371, -0.6576) -> (-14.6742, -0.6576)
  line L491 (-14.2344, -1.5454) -> (-13.371, -1.5454)
  line L492 (-13.371, -1.5454) -> (-13.371, -1.9119)
  line L493 (-13.371, -1.9119) -> (-14.2751, -1.9119)
  line L494 (-14.2751, -1.9119) -> (-14.7676, -1.9119) construction
  line L495 (-14.7676, -1.9119) -> (-15.2036, -1.6351) construction
  line L496 (-15.2036, -1.6351) -> (-15.2036, -0.8938) construction
  spline S34 degree 3 poles (-14.2751, -1.9119) (-14.7676, -1.9119) (-15.2036, -1.6351) (-15.2036, -0.8938) knots 1 1 1 1 2 2 2 2
  line L497 (-15.2036, -0.8938) -> (-15.2036, -0.1491) construction
  line L498 (-15.2036, -0.1491) -> (-14.8923, 0.2057) construction
  line L499 (-14.8923, 0.2057) -> (-14.1529, 0.2057) construction
  spline S35 degree 3 poles (-15.2036, -0.8938) (-15.2036, -0.1491) (-14.8923, 0.2057) (-14.1529, 0.2057) knots 1 1 1 1 2 2 2 2
  line L500 (-14.1529, 0.2057) -> (-13.371, 0.2057)
  line L501 (-13.371, 0.2057) -> (-13.371, -0.169)
  line L502 (-13.371, -0.169) -> (-14.2099, -0.169)
  line L503 (-15.5212, 0.2057) -> (-15.5212, -1.9119)
  line L504 (-15.5212, -1.9119) -> (-15.9855, -1.9119)
  line L505 (-15.9855, -1.9119) -> (-15.9447, -0.2667)
  line L506 (-15.9447, -0.2667) -> (-16.523, -1.9119)
  line L507 (-16.523, -1.9119) -> (-17.0198, -1.9119)
  line L508 (-17.0198, -1.9119) -> (-17.6144, -0.2504)
  line L509 (-17.6144, -0.2504) -> (-17.5655, -1.9119)
  line L510 (-17.5655, -1.9119) -> (-18.0379, -1.9119)
  line L511 (-18.0379, -1.9119) -> (-18.0379, 0.2057)
  line L512 (-18.0379, 0.2057) -> (-17.3538, 0.2057)
  line L513 (-17.3538, 0.2057) -> (-16.7836, -1.4232)
  line L514 (-16.7836, -1.4232) -> (-16.2135, 0.2057)
  line L515 (-16.2135, 0.2057) -> (-15.5212, 0.2057)
  line L516 (-18.5103, -1.9119) -> (-18.5103, 0.2057)
  line L517 (-18.5103, 0.2057) -> (-18.999, 0.2057)
  line L518 (-18.999, 0.2057) -> (-18.999, -1.9119)
  line L519 (-18.999, -1.9119) -> (-18.5103, -1.9119)
  line L520 (-19.9519, -1.9119) -> (-20.4406, -1.9119)
  line L521 (-20.4406, -1.9119) -> (-20.4406, -0.169)
  line L522 (-20.4406, -0.169) -> (-21.1573, -0.169)
  line L523 (-21.1573, -0.169) -> (-21.1573, 0.1975)
  line L524 (-21.1573, 0.1975) -> (-19.227, 0.1975)
  line L525 (-19.227, 0.1975) -> (-19.227, -0.169)
  line L526 (-19.227, -0.169) -> (-19.9519, -0.169)
  line L527 (-19.9519, -0.169) -> (-19.9519, -1.9119)
  ellipse E8 centre (-8.3332, -1.1024) end of major axis (-8.3332, -0.425) minor radius 0.6048
  ellipse E9 centre (-8.3332, -1.1024) end of major axis (-8.3332, -0.2279) minor radius 0.8104 (-7.7186, -0.5324) -> (-7.7186, -1.6725) ccw
  line L528 (-7.7186, -1.9282) -> (-7.7186, -1.6725)
  line L529 (-7.7186, -1.9282) -> (-7.515, -1.9282)
  line L530 (-7.515, -1.9282) -> (-7.515, -0.2667)
  line L531 (-7.515, -0.2667) -> (-7.7186, -0.2667)
  line L532 (-7.7186, -0.2667) -> (-7.7186, -0.5324)
  line L533 (-5.6499, 0.2627) -> (-5.8535, 0.2627)
  line L534 (-5.8535, 0.2627) -> (-5.8535, -0.5324)
  line L535 (-5.6499, -1.9282) -> (-5.6499, 0.2627)
  line L536 (-5.8535, -1.9282) -> (-5.6499, -1.9282)
  line L537 (-5.8535, -1.9282) -> (-5.8535, -1.6725)
  ellipse E10 centre (-6.4681, -1.1024) end of major axis (-6.4681, -0.425) minor radius 0.6048
  ellipse E11 centre (-6.4681, -1.1024) end of major axis (-6.4681, -0.2279) minor radius 0.8104 (-5.8535, -0.5324) -> (-5.8535, -1.6725) ccw
  line L538 (10.0774, 0.2627) -> (9.8738, 0.2627)
  line L539 (9.8738, 0.2627) -> (9.8738, -0.5324)
  line L540 (10.0774, -1.9282) -> (10.0774, 0.2627)
  line L541 (9.8738, -1.9282) -> (10.0774, -1.9282)
  line L542 (9.8738, -1.9282) -> (9.8738, -1.6725)
  ellipse E12 centre (9.2591, -1.1024) end of major axis (9.2591, -0.425) minor radius 0.6048
  ellipse E13 centre (9.2591, -1.1024) end of major axis (9.2591, -0.2279) minor radius 0.8104 (9.8738, -0.5324) -> (9.8738, -1.6725) ccw
  line L543 (3.0486, -2.4332) -> (3.2523, -2.4332)
  line L544 (3.2523, -2.4332) -> (3.2523, -1.6381)
  line L545 (3.0486, -0.2423) -> (3.0486, -2.4332)
  line L546 (3.2523, -0.2423) -> (3.0486, -0.2423)
  line L547 (3.2523, -0.2423) -> (3.2523, -0.498)
  ellipse E14 centre (3.8669, -1.0681) end of major axis (3.8669, -1.7455) minor radius 0.6048
  ellipse E15 centre (3.8669, -1.0681) end of major axis (3.8669, -1.9426) minor radius 0.8104 (3.2523, -1.6381) -> (3.2523, -0.498) ccw
  ellipse E16 centre (5.6557, -1.063) end of major axis (5.6557, -0.1727) minor radius 0.8274 (6.4801, -1.1382) -> (6.4279, -1.3825) ccw
  line L548 (5.0581, -0.959) -> (6.2533, -0.959)
  line L549 (5.0547, -1.1382) -> (6.4801, -1.1382)
  line L550 (6.1889, -1.3825) -> (6.4279, -1.3825)
  ellipse E17 centre (5.6557, -1.063) end of major axis (5.6557, -0.3855) minor radius 0.6048 (6.2533, -0.959) -> (5.0581, -0.959) ccw
  ellipse E18 centre (5.6557, -1.063) end of major axis (5.6557, -0.3855) minor radius 0.6048 (5.0547, -1.1382) -> (6.1889, -1.3825) ccw
  line L551 (7.9891, -1.3831) -> (8.2281, -1.3831)
  ellipse E19 centre (7.4558, -1.0635) end of major axis (7.4558, -0.3861) minor radius 0.6048 (6.8548, -1.1387) -> (7.9891, -1.3831) ccw
  line L552 (6.8582, -0.9595) -> (8.0534, -0.9595)
  ellipse E20 centre (7.4558, -1.0635) end of major axis (7.4558, -0.3861) minor radius 0.6048 (8.0534, -0.9595) -> (6.8582, -0.9595) ccw
  ellipse E21 centre (7.4558, -1.0635) end of major axis (7.4558, -0.1732) minor radius 0.8274 (8.2803, -1.1387) -> (8.2281, -1.3831) ccw
  line L553 (6.8548, -1.1387) -> (8.2803, -1.1387)
  line L554 (15.2819, -4.6893) -> (15.0353, -5.0306) construction
  line L555 (14.1417, -4.7111) -> (14.1417, -4.0784) construction
  spline S36 degree 4 poles (15.2819, -4.6893) (15.0353, -5.0306) (14.3453, -5.0306) (14.1417, -4.7111) (14.1417, -4.0784) knots 1 1 1 1 1 2 2 2 2 2
  line L556 (15.0353, -5.0306) -> (14.3453, -5.0306) construction
  line L557 (14.3453, -5.0306) -> (14.1417, -4.7111) construction
  line L558 (14.3453, -4.0947) -> (14.3453, -4.5665) construction
  line L559 (14.3453, -4.5665) -> (14.6572, -4.7756) construction
  line L560 (14.6572, -4.7756) -> (14.9843, -4.7756) construction
  line L561 (14.9843, -4.7756) -> (15.2819, -4.5319) construction
  line L562 (15.2819, -4.5319) -> (15.2819, -4.1273) construction
  spline S37 degree 4 poles (14.3453, -4.0947) (14.3453, -4.5665) (14.6572, -4.7756) (14.9843, -4.7756) (15.2819, -4.5319) (15.2819, -4.1273) knots 1 1 1 1 1 2 3 3 3 3 3
  line L563 (14.3453, -4.0947) -> (14.3453, -3.2151)
  line L564 (14.3453, -3.2151) -> (14.1417, -3.2151)
  line L565 (14.1417, -3.2151) -> (14.1417, -4.0784)
  line L566 (15.2819, -4.1273) -> (15.2819, -3.2151)
  line L567 (15.2819, -3.2151) -> (15.4856, -3.2151)
  line L568 (15.4856, -3.2151) -> (15.4856, -4.8684)
  line L569 (15.4856, -4.8684) -> (15.2819, -4.8684)
  line L570 (15.2819, -4.8684) -> (15.2819, -4.6893)
  line L571 (17.1634, -11.6122) -> (17.1634, -9.4193)
  line L572 (17.367, -10.2954) -> (17.367, -10.7) construction
  spline S38 degree 4 poles (18.3036, -10.7326) (18.3036, -10.2608) (17.9917, -10.0517) (17.6646, -10.0517) (17.367, -10.2954) (17.367, -10.7) knots 1 1 1 1 1 2 3 3 3 3 3
  line L573 (18.3036, -10.7326) -> (18.3036, -10.2608) construction
  line L574 (18.3036, -10.2608) -> (17.9917, -10.0517) construction
  line L575 (17.9917, -10.0517) -> (17.6646, -10.0517) construction
  line L576 (17.6646, -10.0517) -> (17.367, -10.2954) construction
  line L577 (17.1634, -9.4193) -> (17.367, -9.4193)
  line L578 (17.367, -9.4193) -> (17.367, -10.138)
  line L579 (17.367, -10.138) -> (17.6136, -9.7967) construction
  spline S39 degree 4 poles (17.367, -10.138) (17.6136, -9.7967) (18.3036, -9.7967) (18.5072, -10.1162) (18.5072, -10.7489) knots 1 1 1 1 1 2 2 2 2 2
  line L580 (17.6136, -9.7967) -> (18.3036, -9.7967) construction
  line L581 (18.3036, -9.7967) -> (18.5072, -10.1162) construction
  line L582 (18.5072, -10.1162) -> (18.5072, -10.7489) construction
  line L583 (17.367, -11.6122) -> (17.1634, -11.6122)
  line L584 (17.367, -10.7) -> (17.367, -11.6122)
  line L585 (18.3036, -10.7326) -> (18.3036, -11.6122)
  line L586 (18.5072, -11.6122) -> (18.5072, -10.7489)
  line L587 (18.3036, -11.6122) -> (18.5072, -11.6122)
  line L588 (12.3661, -2.6775) -> (12.5779, -2.6775)
  line L589 (12.5779, -2.6775) -> (12.5779, -3.663)
  line L590 (12.5779, -3.663) -> (13.5797, -3.663)
  line L591 (13.5797, -3.663) -> (13.5797, -2.6775)
  line L592 (13.5797, -2.6775) -> (13.7915, -2.6775)
  line L593 (13.7915, -2.6775) -> (13.7915, -4.8684)
  line L594 (13.7915, -4.8684) -> (13.5797, -4.8684)
  line L595 (13.5797, -4.8684) -> (13.5797, -3.8666)
  line L596 (13.5797, -3.8666) -> (12.5779, -3.8666)
  line L597 (12.5779, -3.8666) -> (12.5779, -4.8684)
  line L598 (12.5779, -4.8684) -> (12.3661, -4.8684)
  line L599 (12.3661, -4.8684) -> (12.3661, -2.6775)
  line L600 (-3.7114, -0.6033) -> (-3.7114, -1.0079) construction
  spline S40 degree 4 poles (-2.7748, -1.0404) (-2.7748, -0.5686) (-3.0867, -0.3596) (-3.4138, -0.3596) (-3.7114, -0.6033) (-3.7114, -1.0079) knots 1 1 1 1 1 2 3 3 3 3 3
  line L601 (-2.7748, -1.0404) -> (-2.7748, -0.5686) construction
  line L602 (-2.7748, -0.5686) -> (-3.0867, -0.3596) construction
  line L603 (-3.0867, -0.3596) -> (-3.4138, -0.3596) construction
  line L604 (-3.4138, -0.3596) -> (-3.7114, -0.6033) construction
  line L605 (-3.4138, -0.1403) -> (-2.9026, -0.1562) construction
  spline S41 degree 3 poles (-3.7114, -0.454) (-3.4138, -0.1403) (-2.9026, -0.1562) (-2.6526, -0.5273) knots 1 1 1 1 2 2 2 2
  line L606 (-3.7114, -0.454) -> (-3.4138, -0.1403) construction
  line L607 (-2.9026, -0.1562) -> (-2.6526, -0.5273) construction
  line L608 (-2.3639, -0.0983) -> (-1.6738, -0.0983) construction
  spline S42 degree 4 poles (-2.6526, -0.5273) (-2.3639, -0.0983) (-1.6738, -0.0983) (-1.4702, -0.4178) (-1.4702, -1.0505) knots 1 1 1 1 1 2 2 2 2 2
  line L609 (-2.6526, -0.5273) -> (-2.3639, -0.0983) construction
  line L610 (-1.6738, -0.0983) -> (-1.4702, -0.4178) construction
  line L611 (-1.4702, -0.4178) -> (-1.4702, -1.0505) construction
  line L612 (-1.9558, -0.3808) -> (-2.2829, -0.3808) construction
  spline S43 degree 4 poles (-1.6671, -1.0404) (-1.6671, -0.5898) (-1.9558, -0.3808) (-2.2829, -0.3808) (-2.5875, -0.5897) (-2.5875, -1.1137) knots 1 1 1 1 1 2 3 3 3 3 3
  line L613 (-1.6671, -1.0404) -> (-1.6671, -0.5898) construction
  line L614 (-1.6671, -0.5898) -> (-1.9558, -0.3808) construction
  line L615 (-2.2829, -0.3808) -> (-2.5875, -0.5897) construction
  line L616 (-2.5875, -0.5897) -> (-2.5875, -1.1137) construction
  line L617 (-3.9151, -1.9201) -> (-3.9151, -0.2667)
  line L618 (-3.7114, -0.2667) -> (-3.7114, -0.454)
  line L619 (-3.9151, -0.2667) -> (-3.7114, -0.2667)
  line L620 (-2.7748, -1.0404) -> (-2.7748, -1.9201)
  line L621 (-1.6671, -1.9201) -> (-1.4702, -1.9201)
  line L622 (-2.5875, -1.9201) -> (-2.7748, -1.9201)
  line L623 (-1.4702, -1.9201) -> (-1.4702, -1.0505)
  line L624 (-1.6671, -1.0404) -> (-1.6671, -1.9201)
  line L625 (-2.5875, -1.1137) -> (-2.5875, -1.9201)